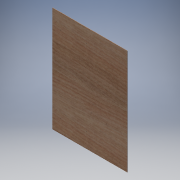
# Autodesk Inventor part: sol
Saved by Autodesk Inventor 2019 (Build 230136000, 136)
## iProperties
Created: 2017-12-27
Part Number: sol
Material: Generic
Document SubType Name: Modeling
Designer: franc
Density: 1 g/cm^3
Appearance: Default
Mass: 87.5 g
Surface Area: 1762 cm^2
Volume: 87.5 cm^3
Author: franc
Autodesk Inventor part; units mm, degrees
ref_plane "YZ Plane" through (0, 0, 0) normal (1, 0, 0) x (0, 1, 0)
ref_plane "XZ Plane" through (0, 0, 0) normal (0, 1, 0) x (-1, 0, 0)
ref_plane "XY Plane" through (0, 0, 0) normal (0, 0, 1) x (1, 0, 0)
sketch "Esquisse1" plane through (0, 0, 0) normal (0, 1, 0) x (-1, 0, 0)
  line L0 (6.5441, 9.8275) -> (-243.4559, 9.8275)
  line L1 (-243.4559, 9.8275) -> (-243.4559, -340.1725)
  line L2 (-243.4559, -340.1725) -> (6.5441, -340.1725)
  line L3 (6.5441, -340.1725) -> (6.5441, 9.8275)
  point P0 (0, 0)
  dimension "d0" = 350
  dimension "d1" = 250
  constraints: 8 end point, 2 parallel, 1 horizontal, 1 perpendicular
  measures "d0" distance of L2.end L0.start
  measures "d1" distance of L0.start L0.end
extrude "Extrusion1" add sketch "Esquisse1" along normal blind 1
